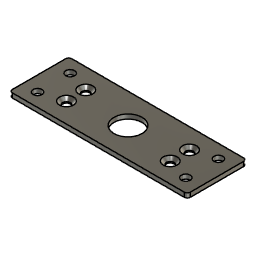
pos14 (Autodesk Fusion 360 design; units mm, degrees)
Autodesk Fusion 360 part; units mm, degrees
sketch "Boceto1" plane through (0, 0, 0) normal (0, 0, 1) x (1, 0, 0)
  line L0 (60, -20) -> (-60, -20)
  line L1 (-60, -20) -> (-60, 20)
  line L2 (-60, 20) -> (60, 20)
  line L3 (60, 20) -> (60, -20)
  line L4 (60, -20) -> (-60, 20) construction
  line L5 (-60, -20) -> (60, 20) construction
  circle A0 centre (0, 0) radius 9.5
  circle A1 centre (-50, 11) radius 3
  circle A2 centre (50, 11) radius 3
  circle A3 centre (-50, -11) radius 3
  circle A4 centre (50, -11) radius 3
  dimension "d1" = 120
  dimension "d2" = 40
  dimension "d3" = 19
  dimension "d4" = 6
  dimension "d5" = 10
  dimension "d6" = 11
  dimension "d9" = 100
  dimension "d10" = -22
  constraint horizontal L0
  constraint perpendicular L0 L1
  constraint parallel L0 L2
  constraint parallel L1 L3
  constraint coincident L4 A0.centre
  constraint coincident L5 A0.centre
  constraint coincident A0.centre origin
  measures "d1" distance of L1.end L2.end
  measures "d2" distance of L0.end L1.end
  measures "d3" diameter of A0
  measures "d4" diameter of A1
  measures "d5" distance of L1 A1.centre
  measures "d6" vertical distance of A0.centre A1.centre
extrude "Extruir1" add sketch "Boceto1" along normal blind 3
sketch "Boceto2" plane through (0, 0, 3) normal (0, 0, 1) x (-1, 0, 0)
  circle A0 centre (0, 0) radius 9.5
  circle A1 centre (-50, -11) radius 3
  circle A2 centre (-50, 11) radius 3
  circle A3 centre (50, -11) radius 3
  circle A4 centre (50, 11) radius 3
  line L0 (-60, -20) -> (60, -20)
  line L1 (60, -20) -> (60, 20)
  line L2 (60, 20) -> (-60, 20)
  line L3 (-60, 20) -> (-60, -20)
  line L4 (35, -6.5) -> (-35, -6.5) construction
  line L5 (-35, -6.5) -> (-35, 6.5) construction
  line L6 (-35, 6.5) -> (35, 6.5) construction
  line L7 (35, 6.5) -> (35, -6.5) construction
  line L8 (35, -6.5) -> (-35, 6.5) construction
  line L9 (-35, -6.5) -> (35, 6.5) construction
  point P0 (35, -6.5)
  point P1 (35, 6.5)
  point P2 (-35, 6.5)
  point P3 (-35, -6.5)
  dimension "d18" = 13
  dimension "d19" = 25
  constraint horizontal L4
  constraint perpendicular L4 L5
  constraint parallel L4 L6
  constraint parallel L5 L7
  constraint coincident L8 A0.centre
  constraint coincident L9 A0.centre
  constraint coincident A0.centre origin
  constraint coincident P0 L4.start
  constraint coincident P1 L6.end
  constraint coincident P2 L5.end
  constraint coincident P3 L4.end
  measures "d18" distance of P0 P1
  measures "d19" distance of L1 L7
hole "Agujero2" at (35, 6.5, 3) at (-35, 6.5, 3) at (-35, -6.5, 3) at (35, -6.5, 3) direction (0, 0, -1) diameter 5.2 depth 15 tip angle 180 countersink diameter 9.5 countersink angle 90
fillet "Empalme1" radius 2 4 edges at (-60, -20, 1.5) (-60, 20, 1.5) (60, -20, 1.5) (60, 20, 1.5)
